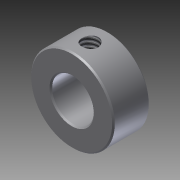
# Autodesk Inventor part: SC-8-F
Saved by Autodesk Inventor 2013 (Build 170138000, 138)
## iProperties
Category: Miscellaneous
Company: Autodesk Inc.
Created: 2012-12-03
Part Number: SC-8-F
Document SubType Name: Modeling
Designer: Autodesk Inc.
Density: 1 g/cm^3
Material: Generic
Author: Autodesk Inc.
Autodesk Inventor part; units mm, degrees
note: some values were not read from the file. Chosen so that the rebuilt part matches the saved one: direction of "Hole1".
ref_plane "YZ Plane" through (0, 0, 0) normal (1, 0, 0) x (0, 1, 0)
ref_plane "XY Plane" through (0, 0, 0) normal (0, 0, 1) x (1, 0, 0)
sketch "Sketch1" plane through (0, 0, 0) normal (0, 0, 1) x (1, 0, 0)
  circle A0 centre (0, 0) radius 12.7
  dimension "d0" = 25.4
  constraints: 1 centre point, 1 coincident
  measures "d0" diameter of A0
extrude "Extrusion1" add sketch "Sketch1" against normal blind 11.1252
sketch "Sketch2" plane through (0, 0, 0) normal (0, 0, 1) x (1, 0, 0)
  circle A0 centre (0, 0) radius 12.7 projected
  circle A1 centre (0, 0) radius 6.35
  dimension "d3" = 12.7
  constraints: 1 centre point, 1 coincident
  measures "d3" diameter of A1
extrude "Extrusion2" cut sketch "Sketch2" against normal up to next contours A1
chamfer "Chamfer1" distance 0.3969 angle 45 4 edges at (-12.7, 0, 0) (-12.7, 0, -11.1252) (-6.35, 0, 0) (-6.35, 0, -11.1252)
ref_plane "Work Plane1" through (0, 12.7, 0) normal (0, 1, 0) x (-1, 0, 0)
sketch "Sketch3" plane through (0, 12.7, 0) normal (0, 1, 0) x (-1, 0, 0)
  line L0 (12.3031, -11.1252) -> (-12.3031, -11.1252) projected
  line L1 (12.7, -0.3969) -> (12.7, -10.7283) projected
  point P0 (0, 0)
  point P1 (0, -5.5626)
  point P2 (0, -11.1252)
  point P3 (12.7, -5.5626)
  constraints: 2 midpoint, 1 horizontal alignment, 1 vertical alignment
hole "Hole1" at (0, 12.7, -5.5626) direction (0, -1, 0) diameter 4.9784 end up to surface thread size "1/4-20 UNC" class "2B" standard "ANSI Unified Screw Threads"
body "Solid1"
